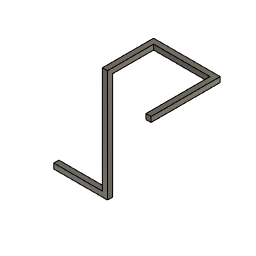
Square_Pipe (Autodesk Fusion 360 design; units mm, degrees)
Autodesk Fusion 360 part; units mm, degrees
sketch "Pipe path" plane through (0, 0, 0) normal (0, 0, 1) x (1, 0, 0)
  line L0 (0, 0) -> (50, 0)
  line L1 (50, 0, 0) -> (50, 0, 104.3203)
  line L2 (50, 0, 104.3203) -> (50, 45, 104.3203)
  line L3 (50, 45, 104.3203) -> (110, 45, 104.3203)
  line L4 (110, 45, 104.3203) -> (110, -20, 104.3203)
  constraint coincident L0.start origin
  constraint horizontal L0
pipe "Pipe1" add square section size 5 path "Pipe path" along L0 L1 L2 L3 L4
named bodies: "Pipe"
